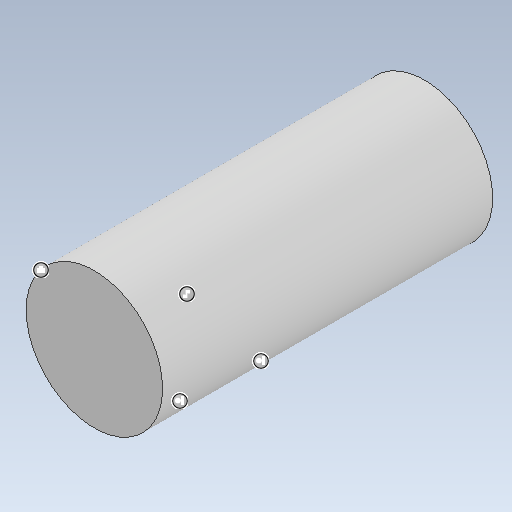
# Autodesk Inventor part: Mold Design Stop Pin
Saved by Autodesk Inventor 2021 (Build 250183000, 183)
## iProperties
Created: 2007-09-05
Part Number: Mold Design Stop Pin
Document SubType Name: Modeling
Designer: mxwang
Density: 1 g/cm^3
Material: Generic
Appearance: Default
Author: mxwang
Autodesk Inventor part; units mm, degrees
ref_plane "YZ Plane" through (0, 0, 0) normal (1, 0, 0) x (0, 1, 0)
ref_plane "XZ Plane" through (0, 0, 0) normal (0, 1, 0) x (-1, 0, 0)
ref_plane "XY Plane" through (0, 0, 0) normal (0, 0, 1) x (1, 0, 0)
sketch "Sketch1" plane through (0, 0, 0) normal (0, 0, 1) x (1, 0, 0)
  circle A0 centre (0, 0) radius 4.1321
  dimension "Diameter" = 8.2642
  constraints: 1 centre point, 1 coincident
  measures "Diameter" diameter of A0
extrude "Extrusion1" add sketch "Sketch1" along normal mid plane 20
body "Solid1"
